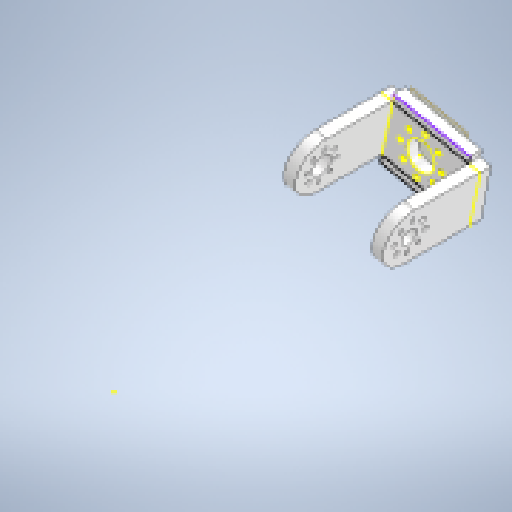
# Autodesk Inventor part: 37
Saved by Autodesk Inventor 2024.3 (Build 283343000, 343)
## iProperties
Created: 2024-09-07
Part Number: 37
Material: LCP 플라스틱
Document SubType Name: Modeling
Designer: 구지현
Density: 1.626 g/cm^3
Appearance: 매끄러움 - 흰색
Mass: 34.2854 g
Surface Area: 107.702 cm^2
Volume: 21.0857 cm^3
Author: 구지현
Autodesk Inventor part; units mm, degrees
ref_plane "YZ Plane" through (0, 0, 0) normal (1, 0, 0) x (0, 1, 0)
ref_plane "XZ Plane" through (0, 0, 0) normal (0, 1, 0) x (-1, 0, 0)
ref_plane "XY Plane" through (0, 0, 0) normal (0, 0, 1) x (1, 0, 0)
ref_plane "작업 평면1" through (0, 0, -188.9899) normal (0, 0, 1) x (-0.9797373, 0.2002869, 0)
sketch "스케치1" plane through (0, 0, -188.9899) normal (0, 0, 1) x (-0.9797373, 0.2002869, 0)
  circle A0 centre (0, 0) radius 13.8 projected
  circle A1 centre (0, 0) radius 7.2 projected
  circle A2 centre (0, -11) radius 1.2813 projected
  circle A3 centre (-7.7782, -7.7782) radius 1.2813 projected
  circle A4 centre (-11, 0) radius 1.2813 projected
  circle A5 centre (-7.7782, 7.7782) radius 1.2813 projected
  circle A6 centre (0, 11) radius 1.2813 projected
  circle A7 centre (7.7782, 7.7782) radius 1.2813 projected
  circle A8 centre (11, 0) radius 1.2813 projected
  circle A9 centre (7.7782, -7.7782) radius 1.2813 projected
  line L0 (-17.5, -17.5) -> (17.5, -17.5)
  line L1 (17.5, -17.5) -> (17.5, 17.5)
  line L2 (17.5, 17.5) -> (-17.5, 17.5)
  line L3 (-17.5, 17.5) -> (-17.5, -17.5)
  line L4 (-17.5, -17.5) -> (17.5, 17.5) construction
  line L5 (17.5, -17.5) -> (-17.5, 17.5) construction
  circle A10 centre (0, 0) radius 7.3
  circle A11 centre (-11, 0) radius 1.3813
  circle A12 centre (-7.7782, 7.7782) radius 1.3813
  circle A13 centre (0, 11) radius 1.3813
  circle A14 centre (7.7782, 7.7782) radius 1.3813
  circle A15 centre (11, 0) radius 1.1813
  circle A16 centre (7.7782, -7.7782) radius 1.3813
  circle A17 centre (0, -11) radius 1.3813
  circle A18 centre (-7.7782, -7.7782) radius 1.3813
  line L6 (17.2724, -17.5) -> (17.2724, -18.1)
  line L7 (17.1076, 17.5) -> (17.1076, 22.85)
  line L8 (17.1076, 17.5) -> (22.4576, 17.5) construction
  line L9 (17.5, 22.85) -> (16.9, 22.85)
  line L10 (16.9, 22.85) -> (16.9, -18.1)
  line L11 (16.9, -18.1) -> (17.5, -18.1)
  line L12 (17.5, -18.1) -> (17.5, 22.85)
  line L13 (17.5, -18.1) -> (-17.5, -18.1)
  line L14 (-17.5, -18.1) -> (-17.5, 22.85)
  line L15 (-17.5, 22.85) -> (17.5, 22.85)
  line L16 (17.5, 22.85) -> (17.5, -18.1)
  line L17 (17.5, 17.5) -> (18.1, 17.5)
  line L18 (18.1, 17.5) -> (18.1, -17.5)
  line L19 (18.1, -17.5) -> (17.5, -17.5)
  line L20 (17.5, -17.5) -> (17.5, 17.5)
  line L21 (-17.5, 17.5) -> (-22.85, 17.5)
  line L22 (-22.85, 17.5) -> (-22.85, 15.9604)
  line L23 (-22.85, 15.9604) -> (-17.5, 15.9604)
  line L24 (-17.5, 15.9604) -> (-17.5, 17.5)
  line L25 (-22.85, 17.5) -> (-17.5, 17.5)
  line L26 (-17.5, 17.5) -> (-17.5, -17.5)
  line L27 (-17.5, -17.5) -> (-22.85, -17.5)
  line L28 (-22.85, -17.5) -> (-22.85, 17.5)
  point P0 (0, 0)
  point P1 (17.5, -17.5)
  point P2 (-17.5, -17.5)
  point P3 (16.9, -18.1)
  point P4 (16.9, 22.85)
  point P5 (-17.5, 17.5)
  point P6 (17.5, 17.5)
  point P7 (-22.85, 15.9604)
  point P8 (17.5, -17.5)
  dimension "d0" = 35
  dimension "d1" = 35
  dimension "d2" = 0.1
  dimension "d3" = 0.1
  dimension "d4" = 0.1
  dimension "d5" = 0.1
  dimension "d6" = 0.1
  dimension "d7" = 0.1
  dimension "d8" = 0.1
  dimension "d9" = 0.1
  dimension "d10" = 0.1
  dimension "d13" = 0.6
  dimension "d14" = 5.35
  dimension "d15" = 90
  dimension "d16" = 0.6
  dimension "d17" = 5.35
  constraints: 58 end point, 12 parallel, 9 centre point, 8 perpendicular, 7 horizontal, 2 midpoint, 2 point on line, 1 vertical
  measures "d0" distance of L2.end L1.end
  measures "d1" distance of L1.end L0.end
  measures "d2" radial gap between concentric circles of A1 A10
  measures "d3" radial gap between concentric circles of A4 A11
  measures "d4" radial gap between concentric circles of A5 A12
  measures "d5" radial gap between concentric circles of A6 A13
  measures "d6" radial gap between concentric circles of A7 A14
  measures "d7" radial gap between concentric circles of A8 A15
  measures "d8" radial gap between concentric circles of A9 A16
  measures "d9" radial gap between concentric circles of A2 A17
  measures "d10" radial gap between concentric circles of A3 A18
  measures "d13" distance of L6.start L6.end
  measures "d14" distance of L7.start L7.end
  measures "d15" angle of L8 L7
  measures "d16" distance of L18.end L19.end
  measures "d17" distance of L23.end L22.end
extrude "돌출1" add sketch "스케치1" along normal blind 6 contours A0 | L0 L10 L2 L1 | L1 L17 L18 L19 | L0 L3 L2 L10 | L27 L28 L23 L3 | L23 L22 L21 L3
sketch "스케치3" plane through (25.892, 12.5688, -182.9899) normal (0.9797373, -0.2002869, 0) x (0, 0, -1)
  circle A0 centre (2.59, -25.3) radius 1.55 projected
  circle A1 centre (2.59, -9.7) radius 1.55 projected
  line L0 (-34, -31.3) -> (6, -31.3) projected
  line L1 (6, -31.3) -> (6, -3.7) projected
  line L2 (6, -3.7) -> (-34, -3.7) projected
  arc A2 (-34, -3.7) -> (-34, -31.3) centre (-34, -17.5) ccw projected
  circle A3 centre (-41.7782, -25.2782) radius 1.65 projected
  circle A4 centre (-45, -17.5) radius 1.65 projected
  circle A5 centre (-41.7782, -9.7218) radius 1.65 projected
  circle A6 centre (-34, -6.5) radius 1.65 projected
  circle A7 centre (-26.2218, -9.7218) radius 1.65 projected
  circle A8 centre (-23, -17.5) radius 1.65 projected
  circle A9 centre (-26.2218, -25.2782) radius 1.65 projected
  circle A10 centre (-34, -28.5) radius 1.65 projected
  circle A11 centre (-34, -17.5) radius 5.1 projected
  circle A12 centre (-34, -17.5) radius 3.9 projected
  circle A13 centre (-34, -17.5) radius 4
  circle A14 centre (-28.3126, -11.8739) radius 1.2 projected
  circle A15 centre (-39.6261, -11.8126) radius 1.2 projected
  circle A16 centre (-39.6874, -23.1261) radius 1.2 projected
  circle A17 centre (-28.3739, -23.1874) radius 1.2 projected
  circle A18 centre (-34, -17.5) radius 4 projected
  circle A19 centre (-34, -17.5) radius 10.9 projected
  circle A20 centre (-34.0433, -25.4999) radius 1.2 projected
  circle A21 centre (-41.9999, -17.4567) radius 1.2 projected
  circle A22 centre (-33.9567, -9.5001) radius 1.2 projected
  circle A23 centre (-26.0001, -17.5433) radius 1.2 projected
  circle A24 centre (-34, -17.5) radius 3.5 projected
  circle A25 centre (-34, -17.5) radius 5.2
  circle A26 centre (-26.0001, -17.5433) radius 1.3
  circle A27 centre (-28.3739, -23.1874) radius 1.3
  circle A28 centre (-34.0433, -25.4999) radius 1.3
  circle A29 centre (-39.6874, -23.1261) radius 1.3
  circle A30 centre (-41.9999, -17.4567) radius 1.3
  circle A31 centre (-39.6261, -11.8126) radius 1.3
  circle A32 centre (-33.9567, -9.5001) radius 1.3
  circle A33 centre (-28.3126, -11.8739) radius 1.3
  point P0 (-182.9899, -17.5)
  dimension "d22" = 0.1
  dimension "d23" = 0.1
  dimension "d24" = 0.1
  dimension "d25" = 0.1
  dimension "d26" = 0.1
  dimension "d27" = 0.1
  dimension "d28" = 0.1
  dimension "d29" = 0.1
  dimension "d30" = 0.1
  dimension "d31" = 0.1
  constraints: 10 centre point
  measures "d22" radial gap between concentric circles of A12 A13
  measures "d23" radial gap between concentric circles of A11 A25
  measures "d24" radial gap between concentric circles of A23 A26
  measures "d25" radial gap between concentric circles of A17 A27
  measures "d26" radial gap between concentric circles of A20 A28
  measures "d27" radial gap between concentric circles of A16 A29
  measures "d28" radial gap between concentric circles of A21 A30
  measures "d29" radial gap between concentric circles of A15 A31
  measures "d30" radial gap between concentric circles of A22 A32
  measures "d31" radial gap between concentric circles of A14 A33
extrude "돌출2" add sketch "스케치3" along normal blind 6 contours A0 | A1 | A2 L2 L1 L0 | A3 A19 | A3 A19 A4 A5 A6 A7 A8 A9 A10 | A19 A3 | A19 A4 | A4 A19 | A19 A10 | A10 A19 | A19 A5 | A5 A19 | A19 A9 | A9 A19 | A19 A6 | A6 A19 | A19 A8 | A8 A19 | A19 A7 | A7 A19 | A11 | A25
sketch "스케치4" plane through (-21.2383, -13.5202, -188.9899) normal (-0.9797373, 0.2002869, 0) x (0, 0, 1)
  circle A0 centre (3.41, 9.7) radius 1.55 projected
  circle A1 centre (3.41, 25.3) radius 1.55 projected
  line L0 (40, 3.7) -> (0, 3.7) projected
  arc A2 (40, 3.7) -> (40, 31.3) centre (40, 17.5) ccw projected
  line L1 (0, 31.3) -> (40, 31.3) projected
  line L2 (0, 3.7) -> (0, 31.3) projected
  circle A3 centre (47.7782, 9.7218) radius 1.65 projected
  circle A4 centre (51, 17.5) radius 1.65 projected
  circle A5 centre (47.7782, 25.2782) radius 1.65 projected
  circle A6 centre (40, 28.5) radius 1.65 projected
  circle A7 centre (32.2218, 25.2782) radius 1.65 projected
  circle A8 centre (29, 17.5) radius 1.65 projected
  circle A9 centre (32.2218, 9.7218) radius 1.65 projected
  circle A10 centre (40, 6.5) radius 1.65 projected
  circle A11 centre (40, 17.5) radius 5.1 projected
  circle A12 centre (40, 17.5) radius 10.8 projected
  circle A13 centre (40, 17.5) radius 6 projected
  circle A14 centre (47.9984, 17.6612) radius 1.05 projected
  circle A15 centre (45.7697, 11.9583) radius 1.05 projected
  circle A16 centre (40.1612, 9.5016) radius 1.05 projected
  circle A17 centre (34.4583, 11.7303) radius 1.05 projected
  circle A18 centre (32.0016, 17.3388) radius 1.05 projected
  circle A19 centre (34.2303, 23.0417) radius 1.05 projected
  circle A20 centre (39.8388, 25.4984) radius 1.05 projected
  circle A21 centre (45.5417, 23.2697) radius 1.05 projected
  circle A22 centre (39.8388, 25.4984) radius 1.15
  circle A23 centre (34.2303, 23.0417) radius 1.15
  circle A24 centre (32.0016, 17.3388) radius 1.15
  circle A25 centre (34.4583, 11.7303) radius 1.15
  circle A26 centre (40.1612, 9.5016) radius 1.15
  circle A27 centre (45.7697, 11.9583) radius 1.15
  circle A28 centre (47.9984, 17.6612) radius 1.15
  circle A29 centre (45.5417, 23.2697) radius 1.15
  point P0 (188.9899, 17.5)
  dimension "d32" = 0.1
  dimension "d33" = 0.1
  dimension "d34" = 0.1
  dimension "d35" = 0.1
  dimension "d36" = 0.1
  dimension "d37" = 0.1
  dimension "d38" = 0.1
  dimension "d39" = 0.1
  constraints: 8 centre point
  measures "d32" radial gap between concentric circles of A20 A22
  measures "d33" radial gap between concentric circles of A19 A23
  measures "d34" radial gap between concentric circles of A18 A24
  measures "d35" radial gap between concentric circles of A17 A25
  measures "d36" radial gap between concentric circles of A16 A26
  measures "d37" radial gap between concentric circles of A15 A27
  measures "d38" radial gap between concentric circles of A14 A28
  measures "d39" radial gap between concentric circles of A21 A29
extrude "돌출3" add sketch "스케치4" along normal blind 6 contours A0 | A1 | L0 L2 L1 A2 | A3 A12 | A12 A3 | A3 A12 A10 A9 A8 A7 A6 A5 A4 | A12 A4 | A4 A12 | A12 A10 | A10 A12 | A12 A5 | A5 A12 | A12 A9 | A9 A12 | A12 A6 | A6 A12 | A12 A8 | A8 A12 | A12 A7 | A7 A12 | A13
sketch "스케치5" plane through (0, 0, -182.9899) normal (0, 0, 1) x (0.9797373, -0.2002869, 0)
  line L0 (22.85, 13.8) -> (22.85, -13.8) projected
  line L1 (22.85, -13.8) -> (28.85, -13.8) projected
  line L2 (28.85, 13.8) -> (28.85, -13.8) projected
  line L3 (22.85, 13.8) -> (28.85, 13.8) projected
  line L4 (-18.1, -13.8) -> (-18.1, 13.8) projected
  line L5 (-18.1, 13.8) -> (-24.1, 13.8) projected
  line L6 (-24.1, -13.8) -> (-24.1, 13.8) projected
  line L7 (-18.1, -13.8) -> (-24.1, -13.8) projected
  line L8 (22.85, -17.5) -> (22.85, -13.8) projected
  line L9 (-18.1, -13.8) -> (-18.1, -17.5) projected
  line L10 (22.85, -13.8) -> (-18.1, -13.8)
  line L11 (-18.1, -13.8) -> (-18.1, -17.5)
  line L12 (-18.1, -17.5) -> (22.85, -17.5)
  line L13 (22.85, -17.5) -> (22.85, -13.8)
  line L14 (-18.1, -17.5) -> (22.85, -17.5) projected
  line L15 (22.85, -17.5) -> (22.85, -13.8) projected
  line L16 (22.85, -13.8) -> (22.85, 13.8) projected
  line L17 (22.85, 13.8) -> (22.85, 17.5) projected
  line L18 (22.85, 17.5) -> (-18.1, 17.5) projected
  line L19 (-18.1, 17.5) -> (-18.1, 13.8) projected
  line L20 (-18.1, 13.8) -> (-18.1, -13.8) projected
  line L21 (-18.1, -13.8) -> (-18.1, -17.5) projected
  circle A0 centre (-11, 0) radius 1.2813 projected
  circle A1 centre (0, 0) radius 7.3 projected
  circle A2 centre (11, 0) radius 1.3813 projected
  circle A3 centre (7.7782, -7.7782) radius 1.3813 projected
  circle A4 centre (0, -11) radius 1.3813 projected
  circle A5 centre (-7.7782, -7.7782) radius 1.3813 projected
  circle A6 centre (-7.7782, 7.7782) radius 1.3813 projected
  circle A7 centre (0, 11) radius 1.3813 projected
  circle A8 centre (7.7782, 7.7782) radius 1.3813 projected
  line L22 (22.85, 13.8) -> (-18.3673, 13.8)
  line L23 (-18.3673, 13.8) -> (-18.3673, 17.5)
  line L24 (-18.3673, 17.5) -> (22.85, 17.5)
  line L25 (22.85, 17.5) -> (22.85, 13.8)
  point P0 (0, 0)
  point P1 (-18.1, 13.8)
  point P2 (-18.1, -13.8)
  point P3 (22.85, -17.5)
  constraints: 16 end point, 4 parallel, 2 horizontal, 2 perpendicular
extrude "돌출4" cut sketch "스케치5" against normal blind 10 contours L22 L19 L18 L17 | L8 L12 L9 L10
